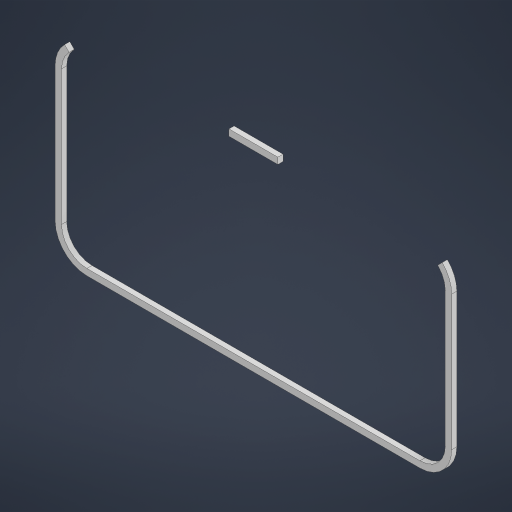
# Autodesk Inventor part: universal_box-seal
Saved by Autodesk Inventor 2024 (Build 280153000, 153)
## iProperties
Created: 2024-03-06
Part Number: universal_box-seal
Material: Všeobecné
Document SubType Name: Modeling
Designer: Simak
Density: 1 g/cm^3
Appearance: Výchozí
Author: Simak
Autodesk Inventor part; units mm, degrees
ref_plane "YZ Plane" through (0, 0, 0) normal (1, 0, 0) x (0, 1, 0)
ref_plane "XZ Plane" through (0, 0, 0) normal (0, 1, 0) x (-1, 0, 0)
ref_plane "XY Plane" through (0, 0, 0) normal (0, 0, 1) x (1, 0, 0)
sketch "Náčrt1" plane through (0, 0, 0) normal (0, 0, 1) x (1, 0, 0)
  line L0 (-42, 25) -> (42, 25)
  line L1 (50, 17) -> (50, -17)
  line L2 (42, -25) -> (-42, -25)
  line L3 (-50, -17) -> (-50, 17)
  line L4 (-50, 25) -> (0, 0) construction
  line L5 (0, 0) -> (50, 25) construction
  line L6 (50, -25) -> (0, 0) construction
  arc A0 (-42, 25) -> (-50, 17) centre (-42, 17) ccw
  arc A1 (-50, -17) -> (-42, -25) centre (-42, -17) ccw
  arc A2 (42, -25) -> (50, -17) centre (42, -17) ccw
  arc A3 (50, 17) -> (42, 25) centre (42, 17) ccw
  line L7 (42, 24.2) -> (-42, 24.2) construction
  arc A4 (-42, 24.2) -> (-49.2, 17) centre (-42, 17) ccw construction
  line L8 (-49.2, 17) -> (-49.2, -17) construction
  arc A5 (-49.2, -17) -> (-42, -24.2) centre (-42, -17) ccw construction
  line L9 (-42, -24.2) -> (42, -24.2) construction
  arc A6 (42, -24.2) -> (49.2, -17) centre (42, -17) ccw construction
  line L10 (49.2, -17) -> (49.2, 17) construction
  arc A7 (49.2, 17) -> (42, 24.2) centre (42, 17) ccw construction
  line L11 (42, -23.4) -> (-42, -23.4)
  arc A8 (-48.4, -17) -> (-42, -23.4) centre (-42, -17) ccw
  line L12 (-48.4, -17) -> (-48.4, 17)
  arc A9 (-42, 23.4) -> (-48.4, 17) centre (-42, 17) ccw
  line L13 (-42, 23.4) -> (42, 23.4)
  arc A10 (48.4, 17) -> (42, 23.4) centre (42, 17) ccw
  line L14 (48.4, 17) -> (48.4, -17)
  arc A11 (42, -23.4) -> (48.4, -17) centre (42, -17) ccw
  line L15 (-42, 26.2) -> (42, 26.2) construction
  arc A12 (51.2, 17) -> (42, 26.2) centre (42, 17) ccw construction
  line L16 (51.2, 17) -> (51.2, -17) construction
  arc A13 (42, -26.2) -> (51.2, -17) centre (42, -17) ccw construction
  line L17 (42, -26.2) -> (-42, -26.2) construction
  arc A14 (-51.2, -17) -> (-42, -26.2) centre (-42, -17) ccw construction
  line L18 (-51.2, -17) -> (-51.2, 17) construction
  arc A15 (-42, 26.2) -> (-51.2, 17) centre (-42, 17) ccw construction
  line L19 (-50, 23.5) -> (50, 23.5) construction
  line L20 (42, 17) -> (47.6134, 22.7)
  line L21 (-42, 17) -> (-47.6134, 22.7)
  line L22 (6.1667, 23.4) -> (6.1667, 26.2)
  line L23 (-6.1667, 23.4) -> (-6.1667, 25)
  point P0 (46.4907, 21.56)
  point P1 (-46.4907, 21.56)
  point P2 (6.1667, 25)
  dimension "d0" = 50
  dimension "d1" = 100
  dimension "d2" = 8
  dimension "d3" = 0.8
  dimension "d4" = 0.8
  dimension "d5" = 2
  dimension "d6" = 2.7
  dimension "d7" = 0.8
  dimension "d8" = 0.8
  dimension "d10" = 35.8333
  dimension "d13" = 35.8333
  constraints: 48 end point, 34 point on circle, 16 centre point, 10 point on line, 9 parallel, 8 tangent, 6 perpendicular, 3 equal radius, 2 equal length, 2 vertical alignment, 1 horizontal, 21 other
  measures "d0" distance of L5.end L6.start
  measures "d1" distance of L4.start L5.end
  measures "d2" radius of A0
  measures "d3" distance between parallel lines of L0 L7
  measures "d4" distance between parallel lines of L9 L11
  measures "d5" distance between parallel lines of L7 L15
  measures "d6" distance between parallel lines of L15 L19
  measures "d7" distance from line of L19 L20.end
  measures "d8" distance from line of L19 L21.end
  measures "d10" distance from line of L13.end L22
  measures "d13" distance from line of L23 L0.start
extrude "Vysunutí1" add sketch "Náčrt1" along normal blind 1.3 contours L0 L22 L13 L23 | L21 A9 L12 A8 L11 A11 L14 A10 L20 A3 L1 A2 L2 A1 L3 A0
equation "\"d4\" = d3"
equation "\"d8\" = d7"
equation "\"d13\" = d10"
